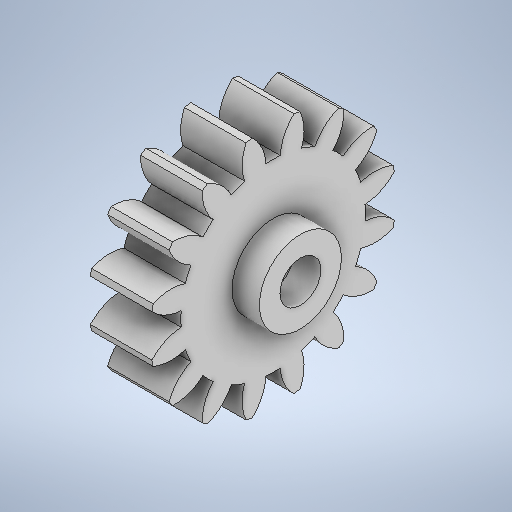
# Autodesk Inventor part: engrane_v3
Saved by Autodesk Inventor 2025.2 (Build 292293000, 293)
## iProperties
Created: 2025-03-05
Part Number: engrane_v3
Material: Generic
Document SubType Name: Modeling
Designer: cdavi
Density: 1 g/cm^3
Appearance: Default
Author: cdavi
Autodesk Inventor part; units mm, degrees
ref_plane "YZ Plane" through (0, 0, 0) normal (1, 0, 0) x (0, 1, 0)
ref_plane "XZ Plane" through (0, 0, 0) normal (0, 1, 0) x (-1, 0, 0)
ref_plane "XY Plane" through (0, 0, 0) normal (0, 0, 1) x (1, 0, 0)
sketch "Sketch1" plane through (0, 0, 0) normal (1, 0, 0) x (0, 1, 0)
  arc A0 (-4.3875, 5.1282) -> (-5.1282, 4.3875) centre (0, 0) ccw
  arc A1 (-5.1895, 7.3532) -> (-4.3875, 5.1282) centre (-1.9912, 7.249) ccw
  arc A2 (-3.0589, 6.016) -> (-4.8075, 7.6084) centre (-5.9352, 4.6137) ccw
  arc A3 (-4.8075, 7.6084) -> (-5.1895, 7.3532) centre (0, 0) ccw
  arc A4 (-2.091, 6.4169) -> (-3.0589, 6.016) centre (0, 0) ccw
  arc A5 (-1.9805, 8.7794) -> (-2.091, 6.4169) centre (0.9345, 7.4592) ccw
  arc A6 (-1.5299, 8.869) -> (-1.9805, 8.7794) centre (0, 0) ccw
  arc A7 (-0.5238, 6.7286) -> (-1.5299, 8.869) centre (-3.7179, 6.5338) ccw
  arc A8 (0.5238, 6.7286) -> (-0.5238, 6.7286) centre (0, 0) ccw
  arc A9 (1.5299, 8.869) -> (0.5238, 6.7286) centre (3.7179, 6.5338) ccw
  arc A10 (1.9805, 8.7794) -> (1.5299, 8.869) centre (0, 0) ccw
  arc A11 (2.091, 6.4169) -> (1.9805, 8.7794) centre (-0.9345, 7.4592) ccw
  arc A12 (3.0589, 6.016) -> (2.091, 6.4169) centre (0, 0) ccw
  arc A13 (4.8075, 7.6084) -> (3.0589, 6.016) centre (5.9352, 4.6137) ccw
  arc A14 (5.1895, 7.3532) -> (4.8075, 7.6084) centre (0, 0) ccw
  arc A15 (4.3875, 5.1282) -> (5.1895, 7.3532) centre (1.9912, 7.249) ccw
  arc A16 (5.1282, 4.3875) -> (4.3875, 5.1282) centre (0, 0) ccw
  arc A17 (7.3532, 5.1895) -> (5.1282, 4.3875) centre (7.249, 1.9912) ccw
  arc A18 (7.6084, 4.8075) -> (7.3532, 5.1895) centre (0, 0) ccw
  arc A19 (6.016, 3.0589) -> (7.6084, 4.8075) centre (4.6137, 5.9352) ccw
  arc A20 (6.4169, 2.091) -> (6.016, 3.0589) centre (0, 0) ccw
  arc A21 (8.7794, 1.9805) -> (6.4169, 2.091) centre (7.4592, -0.9345) ccw
  arc A22 (8.869, 1.5299) -> (8.7794, 1.9805) centre (0, 0) ccw
  arc A23 (6.7286, 0.5238) -> (8.869, 1.5299) centre (6.5338, 3.7179) ccw
  arc A24 (6.7286, -0.5238) -> (6.7286, 0.5238) centre (0, 0) ccw
  arc A25 (8.869, -1.5299) -> (6.7286, -0.5238) centre (6.5338, -3.7179) ccw
  arc A26 (8.7794, -1.9805) -> (8.869, -1.5299) centre (0, 0) ccw
  arc A27 (6.4169, -2.091) -> (8.7794, -1.9805) centre (7.4592, 0.9345) ccw
  arc A28 (6.016, -3.0589) -> (6.4169, -2.091) centre (0, 0) ccw
  arc A29 (7.6084, -4.8075) -> (6.016, -3.0589) centre (4.6137, -5.9352) ccw
  arc A30 (7.3532, -5.1895) -> (7.6084, -4.8075) centre (0, 0) ccw
  arc A31 (5.1282, -4.3875) -> (7.3532, -5.1895) centre (7.249, -1.9912) ccw
  arc A32 (4.3875, -5.1282) -> (5.1282, -4.3875) centre (0, 0) ccw
  arc A33 (5.1895, -7.3532) -> (4.3875, -5.1282) centre (1.9912, -7.249) ccw
  arc A34 (4.8075, -7.6084) -> (5.1895, -7.3532) centre (0, 0) ccw
  arc A35 (3.0589, -6.016) -> (4.8075, -7.6084) centre (5.9352, -4.6137) ccw
  arc A36 (-8.869, 1.5299) -> (-6.7286, 0.5238) centre (-6.5338, 3.7179) ccw
  arc A37 (-6.7286, 0.5238) -> (-6.7286, -0.5238) centre (0, 0) ccw
  arc A38 (-6.7286, -0.5238) -> (-8.869, -1.5299) centre (-6.5338, -3.7179) ccw
  arc A39 (-8.869, -1.5299) -> (-8.7794, -1.9805) centre (0, 0) ccw
  arc A40 (-8.7794, -1.9805) -> (-6.4169, -2.091) centre (-7.4592, 0.9345) ccw
  arc A41 (-6.4169, -2.091) -> (-6.016, -3.0589) centre (0, 0) ccw
  arc A42 (-6.016, -3.0589) -> (-7.6084, -4.8075) centre (-4.6137, -5.9352) ccw
  arc A43 (-7.6084, -4.8075) -> (-7.3532, -5.1895) centre (0, 0) ccw
  arc A44 (-7.3532, -5.1895) -> (-5.1282, -4.3875) centre (-7.249, -1.9912) ccw
  arc A45 (-5.1282, -4.3875) -> (-4.3875, -5.1282) centre (0, 0) ccw
  arc A46 (-4.3875, -5.1282) -> (-5.1895, -7.3532) centre (-1.9912, -7.249) ccw
  arc A47 (-5.1895, -7.3532) -> (-4.8075, -7.6084) centre (0, 0) ccw
  arc A48 (-4.8075, -7.6084) -> (-3.0589, -6.016) centre (-5.9352, -4.6137) ccw
  arc A49 (-3.0589, -6.016) -> (-2.091, -6.4169) centre (0, 0) ccw
  arc A50 (-2.091, -6.4169) -> (-1.9805, -8.7794) centre (0.9345, -7.4592) ccw
  arc A51 (-1.9805, -8.7794) -> (-1.5299, -8.869) centre (0, 0) ccw
  arc A52 (-1.5299, -8.869) -> (-0.5238, -6.7286) centre (-3.7179, -6.5338) ccw
  arc A53 (-0.5238, -6.7286) -> (0.5238, -6.7286) centre (0, 0) ccw
  arc A54 (0.5238, -6.7286) -> (1.5299, -8.869) centre (3.7179, -6.5338) ccw
  arc A55 (1.5299, -8.869) -> (1.9805, -8.7794) centre (0, 0) ccw
  arc A56 (1.9805, -8.7794) -> (2.091, -6.4169) centre (-0.9345, -7.4592) ccw
  arc A57 (2.091, -6.4169) -> (3.0589, -6.016) centre (0, 0) ccw
  arc A58 (3.0589, -6.016) -> (4.8075, -7.6084) centre (5.9352, -4.6137) ccw
  arc A59 (4.8075, -7.6084) -> (5.1895, -7.3532) centre (0, 0) ccw
  arc A60 (5.1895, -7.3532) -> (4.3875, -5.1282) centre (1.9912, -7.249) ccw
  arc A61 (4.3875, -5.1282) -> (5.1282, -4.3875) centre (0, 0) ccw
  arc A62 (5.1282, -4.3875) -> (7.3532, -5.1895) centre (7.249, -1.9912) ccw
  arc A63 (7.3532, -5.1895) -> (7.6084, -4.8075) centre (0, 0) ccw
  arc A64 (7.6084, -4.8075) -> (6.016, -3.0589) centre (4.6137, -5.9352) ccw
  arc A65 (6.016, -3.0589) -> (6.4169, -2.091) centre (0, 0) ccw
  arc A66 (6.4169, -2.091) -> (8.7794, -1.9805) centre (7.4592, 0.9345) ccw
  arc A67 (8.7794, -1.9805) -> (8.869, -1.5299) centre (0, 0) ccw
  arc A68 (8.869, -1.5299) -> (6.7286, -0.5238) centre (6.5338, -3.7179) ccw
  arc A69 (6.7286, -0.5238) -> (6.7286, 0.5238) centre (0, 0) ccw
  arc A70 (6.7286, 0.5238) -> (8.869, 1.5299) centre (6.5338, 3.7179) ccw
  arc A71 (8.869, 1.5299) -> (8.7794, 1.9805) centre (0, 0) ccw
  arc A72 (8.7794, 1.9805) -> (6.4169, 2.091) centre (7.4592, -0.9345) ccw
  arc A73 (6.4169, 2.091) -> (6.016, 3.0589) centre (0, 0) ccw
  arc A74 (6.016, 3.0589) -> (7.6084, 4.8075) centre (4.6137, 5.9352) ccw
  arc A75 (7.6084, 4.8075) -> (7.3532, 5.1895) centre (0, 0) ccw
  arc A76 (7.3532, 5.1895) -> (5.1282, 4.3875) centre (7.249, 1.9912) ccw
  arc A77 (5.1282, 4.3875) -> (4.3875, 5.1282) centre (0, 0) ccw
  arc A78 (4.3875, 5.1282) -> (5.1895, 7.3532) centre (1.9912, 7.249) ccw
  arc A79 (5.1895, 7.3532) -> (4.8075, 7.6084) centre (0, 0) ccw
  arc A80 (4.8075, 7.6084) -> (3.0589, 6.016) centre (5.9352, 4.6137) ccw
  arc A81 (3.0589, 6.016) -> (2.091, 6.4169) centre (0, 0) ccw
  arc A82 (2.091, 6.4169) -> (1.9805, 8.7794) centre (-0.9345, 7.4592) ccw
  arc A83 (1.9805, 8.7794) -> (1.5299, 8.869) centre (0, 0) ccw
  arc A84 (1.5299, 8.869) -> (0.5238, 6.7286) centre (3.7179, 6.5338) ccw
  arc A85 (0.5238, 6.7286) -> (-0.5238, 6.7286) centre (0, 0) ccw
  arc A86 (-0.5238, 6.7286) -> (-1.5299, 8.869) centre (-3.7179, 6.5338) ccw
  arc A87 (-1.5299, 8.869) -> (-1.9805, 8.7794) centre (0, 0) ccw
  arc A88 (-1.9805, 8.7794) -> (-2.091, 6.4169) centre (0.9345, 7.4592) ccw
  arc A89 (-2.091, 6.4169) -> (-3.0589, 6.016) centre (0, 0) ccw
  arc A90 (-3.0589, 6.016) -> (-4.8075, 7.6084) centre (-5.9352, 4.6137) ccw
  arc A91 (-4.8075, 7.6084) -> (-5.1895, 7.3532) centre (0, 0) ccw
  arc A92 (-5.1895, 7.3532) -> (-4.3875, 5.1282) centre (-1.9912, 7.249) ccw
  arc A93 (-4.3875, 5.1282) -> (-5.1282, 4.3875) centre (0, 0) ccw
  arc A94 (-5.1282, 4.3875) -> (-7.3532, 5.1895) centre (-7.249, 1.9912) ccw
  arc A95 (-7.3532, 5.1895) -> (-7.6084, 4.8075) centre (0, 0) ccw
  arc A96 (-7.6084, 4.8075) -> (-6.016, 3.0589) centre (-4.6137, 5.9352) ccw
  arc A97 (-6.016, 3.0589) -> (-6.4169, 2.091) centre (0, 0) ccw
  arc A98 (-6.4169, 2.091) -> (-8.7794, 1.9805) centre (-7.4592, -0.9345) ccw
  arc A99 (-8.7794, 1.9805) -> (-8.869, 1.5299) centre (0, 0) ccw
  circle A100 centre (0, 0) radius 2.5
  line L0 (0, 0) -> (2.25, 0)
  line L1 (-1.5245, 0) -> (0, 0)
  line L2 (0, 0) -> (0, -2.5981)
  point P0 (3.0589, -6.016)
  point P1 (-5.1282, 4.3875)
  dimension "d17" = 5
  constraints: 200 point on circle, 101 centre point, 6 end point, 2 coincident, 1 horizontal, 1 vertical
  measures "d17" diameter of A100
extrude "Extrusion1" add sketch "Sketch1" along normal blind 4.5
sketch "Sketch4" plane through (4.5, 0, 0) normal (1, 0, 0) x (0, 0, -1)
  circle A0 centre (0, 0) radius 1.5
  arc A1 (6.016, 3.0589) -> (7.6084, 4.8075) centre (4.6137, 5.9352) ccw projected
  arc A2 (7.6084, 4.8075) -> (7.3532, 5.1895) centre (0, 0) ccw projected
  arc A3 (7.3532, 5.1895) -> (5.1282, 4.3875) centre (7.249, 1.9912) ccw projected
  arc A4 (5.1282, 4.3875) -> (4.3875, 5.1282) centre (0, 0) ccw projected
  arc A5 (4.3875, 5.1282) -> (5.1895, 7.3532) centre (1.9912, 7.249) ccw projected
  arc A6 (5.1895, 7.3532) -> (4.8075, 7.6084) centre (0, 0) ccw projected
  arc A7 (4.8075, 7.6084) -> (3.0589, 6.016) centre (5.9352, 4.6137) ccw projected
  arc A8 (3.0589, 6.016) -> (2.091, 6.4169) centre (0, 0) ccw projected
  arc A9 (2.091, 6.4169) -> (1.9805, 8.7794) centre (-0.9345, 7.4592) ccw projected
  arc A10 (1.9805, 8.7794) -> (1.5299, 8.869) centre (0, 0) ccw projected
  arc A11 (1.5299, 8.869) -> (0.5238, 6.7286) centre (3.7179, 6.5338) ccw projected
  arc A12 (0.5238, 6.7286) -> (-0.5238, 6.7286) centre (0, 0) ccw projected
  arc A13 (-0.5238, 6.7286) -> (-1.5299, 8.869) centre (-3.7179, 6.5338) ccw projected
  arc A14 (-1.5299, 8.869) -> (-1.9805, 8.7794) centre (0, 0) ccw projected
  arc A15 (-1.9805, 8.7794) -> (-2.091, 6.4169) centre (0.9345, 7.4592) ccw projected
  arc A16 (-2.091, 6.4169) -> (-3.0589, 6.016) centre (0, 0) ccw projected
  arc A17 (-3.0589, 6.016) -> (-4.8075, 7.6084) centre (-5.9352, 4.6137) ccw projected
  arc A18 (-4.8075, 7.6084) -> (-5.1895, 7.3532) centre (0, 0) ccw projected
  arc A19 (-5.1895, 7.3532) -> (-4.3875, 5.1282) centre (-1.9912, 7.249) ccw projected
  arc A20 (-4.3875, 5.1282) -> (-5.1282, 4.3875) centre (0, 0) ccw projected
  arc A21 (-5.1282, 4.3875) -> (-7.3532, 5.1895) centre (-7.249, 1.9912) ccw projected
  arc A22 (-7.3532, 5.1895) -> (-7.6084, 4.8075) centre (0, 0) ccw projected
  arc A23 (-7.6084, 4.8075) -> (-6.016, 3.0589) centre (-4.6137, 5.9352) ccw projected
  arc A24 (-6.016, 3.0589) -> (-6.4169, 2.091) centre (0, 0) ccw projected
  arc A25 (-6.4169, 2.091) -> (-8.7794, 1.9805) centre (-7.4592, -0.9345) ccw projected
  arc A26 (-8.7794, 1.9805) -> (-8.869, 1.5299) centre (0, 0) ccw projected
  arc A27 (-8.869, 1.5299) -> (-6.7286, 0.5238) centre (-6.5338, 3.7179) ccw projected
  arc A28 (-6.7286, 0.5238) -> (-6.7286, -0.5238) centre (0, 0) ccw projected
  arc A29 (-6.7286, -0.5238) -> (-8.869, -1.5299) centre (-6.5338, -3.7179) ccw projected
  arc A30 (-8.869, -1.5299) -> (-8.7794, -1.9805) centre (0, 0) ccw projected
  arc A31 (-8.7794, -1.9805) -> (-6.4169, -2.091) centre (-7.4592, 0.9345) ccw projected
  arc A32 (-6.4169, -2.091) -> (-6.016, -3.0589) centre (0, 0) ccw projected
  arc A33 (-6.016, -3.0589) -> (-7.6084, -4.8075) centre (-4.6137, -5.9352) ccw projected
  arc A34 (-7.6084, -4.8075) -> (-7.3532, -5.1895) centre (0, 0) ccw projected
  arc A35 (-7.3532, -5.1895) -> (-5.1282, -4.3875) centre (-7.249, -1.9912) ccw projected
  arc A36 (-5.1282, -4.3875) -> (-4.3875, -5.1282) centre (0, 0) ccw projected
  arc A37 (-4.3875, -5.1282) -> (-5.1895, -7.3532) centre (-1.9912, -7.249) ccw projected
  arc A38 (-5.1895, -7.3532) -> (-4.8075, -7.6084) centre (0, 0) ccw projected
  arc A39 (-4.8075, -7.6084) -> (-3.0589, -6.016) centre (-5.9352, -4.6137) ccw projected
  arc A40 (-3.0589, -6.016) -> (-2.091, -6.4169) centre (0, 0) ccw projected
  arc A41 (-2.091, -6.4169) -> (-1.9805, -8.7794) centre (0.9345, -7.4592) ccw projected
  arc A42 (-1.9805, -8.7794) -> (-1.5299, -8.869) centre (0, 0) ccw projected
  arc A43 (-1.5299, -8.869) -> (-0.5238, -6.7286) centre (-3.7179, -6.5338) ccw projected
  arc A44 (-0.5238, -6.7286) -> (0.5238, -6.7286) centre (0, 0) ccw projected
  arc A45 (0.5238, -6.7286) -> (1.5299, -8.869) centre (3.7179, -6.5338) ccw projected
  arc A46 (1.5299, -8.869) -> (1.9805, -8.7794) centre (0, 0) ccw projected
  arc A47 (1.9805, -8.7794) -> (2.091, -6.4169) centre (-0.9345, -7.4592) ccw projected
  arc A48 (2.091, -6.4169) -> (3.0589, -6.016) centre (0, 0) ccw projected
  arc A49 (3.0589, -6.016) -> (4.8075, -7.6084) centre (5.9352, -4.6137) ccw projected
  arc A50 (4.8075, -7.6084) -> (5.1895, -7.3532) centre (0, 0) ccw projected
  arc A51 (5.1895, -7.3532) -> (4.3875, -5.1282) centre (1.9912, -7.249) ccw projected
  arc A52 (4.3875, -5.1282) -> (5.1282, -4.3875) centre (0, 0) ccw projected
  arc A53 (5.1282, -4.3875) -> (7.3532, -5.1895) centre (7.249, -1.9912) ccw projected
  arc A54 (7.3532, -5.1895) -> (7.6084, -4.8075) centre (0, 0) ccw projected
  arc A55 (7.6084, -4.8075) -> (6.016, -3.0589) centre (4.6137, -5.9352) ccw projected
  arc A56 (6.016, -3.0589) -> (6.4169, -2.091) centre (0, 0) ccw projected
  arc A57 (6.4169, -2.091) -> (8.7794, -1.9805) centre (7.4592, 0.9345) ccw projected
  arc A58 (8.7794, -1.9805) -> (8.869, -1.5299) centre (0, 0) ccw projected
  arc A59 (8.869, -1.5299) -> (6.7286, -0.5238) centre (6.5338, -3.7179) ccw projected
  arc A60 (6.7286, -0.5238) -> (6.7286, 0.5238) centre (0, 0) ccw projected
  arc A61 (6.7286, 0.5238) -> (8.869, 1.5299) centre (6.5338, 3.7179) ccw projected
  arc A62 (8.869, 1.5299) -> (8.7794, 1.9805) centre (0, 0) ccw projected
  arc A63 (8.7794, 1.9805) -> (6.4169, 2.091) centre (7.4592, -0.9345) ccw projected
  arc A64 (6.4169, 2.091) -> (6.016, 3.0589) centre (0, 0) ccw projected
  circle A65 centre (0, 0) radius 2.5 projected
  circle A66 centre (0, 0) radius 3
  dimension "d18" = 3
  dimension "d19" = 6
  constraints: 2 centre point, 2 coincident
  measures "d18" diameter of A0
  measures "d19" diameter of A66
extrude "Extrusion3" add sketch "Sketch4" along normal blind 2 contours A65 | A66
equation "\"d17\" = d_agu"
equation "\"d_agu\" = 5"
body "Solid1"
